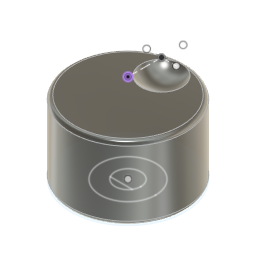
knob_spinner (Autodesk Fusion 360 design; units mm, degrees)
Autodesk Fusion 360 part; units mm, degrees
sketch "Sketch1" plane through (0, 0, 0) normal (0, 0, 1) x (1, 0, 0)
  circle A0 centre (0, 0) radius 14.5
  dimension "d1" = 29
  constraint coincident A0.centre origin
  measures "d1" diameter of A0
extrude "Extrude1" add sketch "Sketch1" along normal blind 18.5
sketch "Sketch2" plane through (0, 0, 0) normal (0, 0, -1) x (1, 0, 0)
  circle A0 centre (0, 0) radius 14.5
  circle A1 centre (0, 0) radius 7
  circle A2 centre (0, 0) radius 3.25
  line L0 (-2.7699, 1.7) -> (2.7699, 1.7)
  dimension "d4" = 14
  dimension "d5" = 1.7
  dimension "d6" = 6.5
  constraint concentric A0 A1
  constraint concentric A1 A2
  constraint coincident A2 L0.start
  constraint coincident A2 L0.end
  constraint horizontal L0
  measures "d4" diameter of A1
  measures "d5" distance of A0.centre L0
  measures "d6" diameter of A2
extrude "Extrude2" cut sketch "Sketch2" against normal blind 18 contours A2 L0 picked at (-0.7022, 0.2404)
extrude "Extrude3" cut sketch "Sketch2" against normal blind 7 contours A2 L0 picked at (-0.7983, 2.2791)
extrude "Extrude4" cut sketch "Sketch2" against normal blind 5 contours A1
fillet "Fillet1" radius 0.5 1 edges at (0, -1.7, 7)
fillet "Fillet1" radius 0.5 1 edges at (-3.0301, 1.1753, 5)
fillet "Fillet1" radius 0.5 1 edges at (-6.5263, -2.5313, 5)
fillet "Fillet2" radius 0.5 1 edges at (-6.5263, -2.5313, 0)
fillet "Fillet3" radius 1 2 edges at (-13.5187, -5.2434, 0) (-13.5187, -5.2434, 18.5)
ref_plane "WorkPlane1" through (0, 0, 22.5) normal (0, 0, 1) x (1, 0, 0)
sketch "Sketch4" plane through (0, 0, 22.5) normal (0, 0, 1) x (1, 0, 0)
  line L0 (0, 0) -> (0, 14) construction
  line L1 (-3.75, 8.5) -> (3.75, 8.5) construction
  point P0 (0, 8.5)
  dimension "d24" = 8.5
  constraint coincident L0.start origin
  constraint vertical L0
  constraint horizontal L1
  constraint midpoint L1 P0
  constraint coincident L0 P0
  measures "d24" distance of L1 L0.start
sphere "SpherePrimitive3" cut diameter 13 placed x (1, 0, 0) y (0, 1, 0) z (0, 0, 1) at (0, 8.5, 22.5)
named bodies: "finger_knob"
